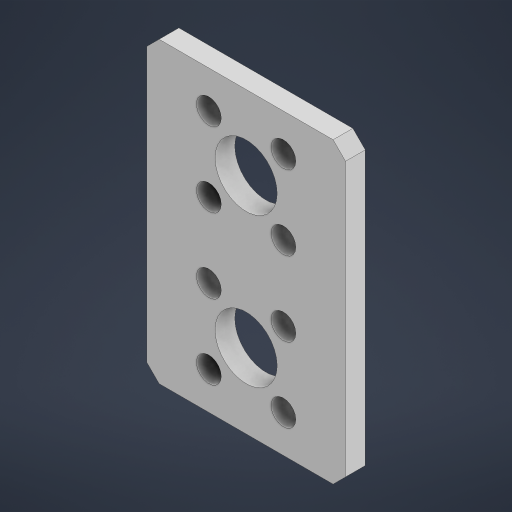
# Autodesk Inventor part: UpperLayerSupportPlate
Saved by Autodesk Inventor 2024 (Build 280153000, 153)
## iProperties
Created: 2023-10-18
Part Number: UpperLayerSupportPlate
Material: Generic
Document SubType Name: Modeling
Designer: avsar
Density: 1 g/cm^3
Appearance: Default
Author: avsar
Autodesk Inventor part; units mm, degrees
ref_plane "YZ Plane" through (0, 0, 0) normal (1, 0, 0) x (0, 1, 0)
ref_plane "XZ Plane" through (0, 0, 0) normal (0, 1, 0) x (-1, 0, 0)
ref_plane "XY Plane" through (0, 0, 0) normal (0, 0, 1) x (1, 0, 0)
sketch "Sketch1" plane through (0, 0, 0) normal (0, 0, 1) x (1, 0, 0)
  line L0 (-16, -24) -> (16, -24)
  line L1 (16, -24) -> (16, 24)
  line L2 (16, 24) -> (-16, 24)
  line L3 (-16, 24) -> (-16, -24)
  line L4 (-16, -24) -> (16, 24) construction
  line L5 (16, -24) -> (-16, 24) construction
  point P0 (0, 0)
  dimension "d0" = 32
  dimension "d1" = 48
  constraints: 12 end point, 2 midpoint, 2 parallel, 1 horizontal, 1 perpendicular
  measures "d0" distance of L2.end L1.end
  measures "d1" distance of L1.end L0.end
extrude "Extrusion1" add sketch "Sketch1" along normal blind 3.175
sketch "Sketch2" plane through (0, 0, 3.175) normal (0, 0, 1) x (1, 0, 0)
  circle A0 centre (0, -12) radius 5
  line L0 (-16, 24) -> (-16, -24) construction
  line L1 (-16, 0) -> (16, 0) construction
  line L2 (16, -24) -> (16, 24) construction
  circle A1 centre (-6, -6) radius 2
  circle A2 centre (-6, -18) radius 2
  circle A3 centre (6, -18) radius 2
  circle A4 centre (6, -6) radius 2
  circle A5 centre (0, 12) radius 5
  circle A6 centre (-6, 6) radius 2
  circle A7 centre (-6, 18) radius 2
  circle A8 centre (6, 18) radius 2
  circle A9 centre (6, 6) radius 2
  point P0 (0, 0)
  dimension "d4" = 10
  dimension "d5" = 12
  dimension "d6" = 4
  dimension "d7" = 6
  dimension "d8" = 6
  dimension "d11" = 360
  constraints: 10 centre point, 5 symmetric about line, 2 end point, 2 midpoint, 1 vertical alignment, 14 other
  measures "d4" diameter of A0
  measures "d5" distance of point (0, 0) A0.centre
  measures "d6" diameter of A1
  measures "d7" horizontal distance of A0.centre A1.centre
  measures "d8" horizontal distance of A1.centre A0.centre
extrude "Extrusion2" cut sketch "Sketch2" against normal through all
chamfer "Chamfer1" distance 2 angle 45 4 edges at (16, 24, 1.5875) (-16, 24, 1.5875) (16, -24, 1.5875) (-16, -24, 1.5875)
body "Solid1"
